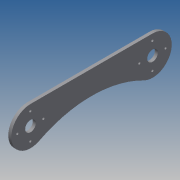
# Autodesk Inventor part: tibia extrude
Saved by Autodesk Inventor 2014 (Build 180170000, 170)
## iProperties
Created: 2015-01-13
Part Number: tibia extrude
Material: Generic
Document SubType Name: Modeling
Designer: I Was ME
Density: 1 g/cm^3
Appearance: Default
Author: I Was ME
Autodesk Inventor part; units mm, degrees
ref_plane "YZ Plane" through (0, 0, 0) normal (1, 0, 0) x (0, 1, 0)
ref_plane "XZ Plane" through (0, 0, 0) normal (0, 1, 0) x (-1, 0, 0)
ref_plane "XY Plane" through (0, 0, 0) normal (0, 0, 1) x (1, 0, 0)
sketch "Sketch1" plane through (0, 0, 0) normal (1, 0, 0) x (0, 1, 0)
  line L0 (-39.75, 25) -> (39.75, 25)
  arc A0 (-39.75, 25) -> (-39.75, 0) centre (-39.75, 12.5) ccw
  arc A1 (39.75, 0) -> (39.75, 25) centre (39.75, 12.5) ccw
  circle A2 centre (39.75, 12.5) radius 3.5
  circle A3 centre (39.75, 21) radius 0.75
  circle A4 centre (48.25, 12.5) radius 0.75
  circle A5 centre (39.75, 4) radius 0.75
  circle A6 centre (31.25, 12.5) radius 0.75
  circle A7 centre (-39.75, 12.5) radius 3.5
  circle A8 centre (-48.25, 12.5) radius 0.75
  circle A9 centre (-39.75, 21) radius 0.75
  circle A10 centre (-31.25, 12.5) radius 0.75
  circle A11 centre (-39.75, 4) radius 0.75
  arc A12 (34.0354, 1.3827) -> (-34.0354, 1.3827) centre (0, -64.8302) ccw
  arc A13 (-39.75, 0) -> (-34.0354, 1.3827) centre (-39.75, 12.5) ccw
  arc A14 (34.0354, 1.3827) -> (39.75, 0) centre (39.75, 12.5) ccw
  point P0 (0, 0)
  point P1 (0, 0)
  dimension "d0" = 79.5
  dimension "d1" = 25
  dimension "d2" = 25
  dimension "d3" = 7
  dimension "d4" = 1.5
  dimension "d5" = 1.5
  dimension "d6" = 1.5
  dimension "d7" = 8.5
  dimension "d8" = 8.5
  dimension "d9" = 8.5
  dimension "d10" = 1.5
  dimension "d11" = 8.5
  dimension "d12" = 7
  dimension "d13" = 1.5
  dimension "d14" = 1.5
  dimension "d15" = 1.5
  dimension "d16" = 1.5
  dimension "d17" = 8.5
  dimension "d18" = 8.5
  dimension "d19" = 8.5
  dimension "d20" = 8.5
  constraints: 15 centre point, 10 point on circle, 6 tangent, 2 coincident, 2 end point, 1 horizontal
  measures "d0" distance of L0.start L0.end
  measures "d1" diameter of A0
  measures "d2" diameter of A1
  measures "d3" diameter of A2
  measures "d4" diameter of A3
  measures "d5" diameter of A4
  measures "d6" diameter of A5
  measures "d7" distance of A1.centre A5.centre
  measures "d8" distance of A1.centre A4.centre
  measures "d9" distance of A1.centre A3.centre
  measures "d10" diameter of A6
  measures "d11" distance of A1.centre A6.centre
  measures "d12" diameter of A7
  measures "d13" diameter of A8
  measures "d14" diameter of A11
  measures "d15" diameter of A10
  measures "d16" diameter of A9
  measures "d17" distance of A0.centre A9.centre
  measures "d18" distance of A0.centre A10.centre
  measures "d19" distance of A0.centre A8.centre
  measures "d20" distance of A11.centre A0.centre
extrude "Extrusion1" add sketch "Sketch1" along normal blind 2
body "Solid1"
